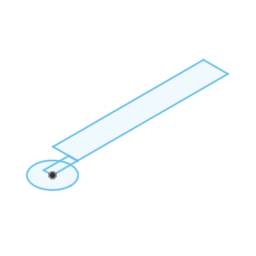
Clip v3 (Autodesk Fusion 360 design; units mm, degrees)
Autodesk Fusion 360 part; units mm, degrees
note: some values were not read from the file. Set by a fixed rule: which sketch regions a step uses.
sketch "Sketch1" plane through (0, 0, 0) normal (0, 0, 1) x (1, 0, 0)
  line L0 (-12.975, 51.3784) -> (12.425, 51.3784)
  line L1 (12.425, 51.3784) -> (12.425, -50.2216)
  line L2 (12.425, -50.2216) -> (-12.975, -50.2216)
  line L3 (-12.975, -50.2216) -> (-12.975, 51.3784)
  line L4 (-0.275, 51.3784) -> (-0.275, -50.2216)
  circle A0 centre (-0.275, -37.535) radius 12.6866
  dimension "d1" = 25.4
  dimension "d2" = 101.6
  constraint horizontal L0
  constraint vertical L1
  constraint horizontal L2
  constraint vertical L3
  constraint midpoint L0 L4.start
  constraint midpoint L2 L4.end
  constraint coincident L4 A0.centre
  constraint coincident L4.end A0
  measures "d1" distance of L0.start L0.end
  measures "d2" distance of L0.start L2.end
extrude "Extrude1" add sketch "Sketch1" along normal blind 25.4 contours L0 L1 L2 L4 A0 | L4 A0 | L4 A0 makes body 1
sketch "Sketch2" plane through (0, 0, 0) normal (0, 0, 1) x (1, 0, 0)
  line L0 (-12.6711, 51.3224) -> (-0.3089, 51.3224)
  line L1 (-0.3089, 51.3224) -> (-0.3089, -24.9086)
  line L2 (-0.3089, -24.9086) -> (-12.6711, -24.9086)
  line L3 (-12.6711, -24.9086) -> (-12.6711, 51.3224)
  circle A0 centre (-0.2821, -37.5504) radius 9.1745
  line L4 (-4.7108, -24.9086) -> (-0.2821, -24.9086)
  line L5 (-0.2821, -24.9086) -> (-0.2821, -37.5504)
  line L6 (-0.2821, -37.5504) -> (-4.7108, -37.5504)
  line L7 (-4.7108, -37.5504) -> (-4.7108, -24.9086)
  constraint horizontal L0
  constraint vertical L1
  constraint horizontal L2
  constraint vertical L3
  constraint horizontal L4
  constraint vertical L5
  constraint horizontal L6
  constraint vertical L7
  constraint coincident A0.centre L5.end
  constraint coincident L2 L4.start
extrude "Extrude2" add sketch "Sketch2" along normal blind 25.4 separate body makes body 2
extrude "Extrude3" cut sketch "Sketch2" along normal blind 261.62 contours A0 L5 L6 L7 | A0 L5 L6 L7 bodies 1
sketch "Sketch3" plane through (0, 0, 25.4) normal (0, 0, 1) x (-1, 0, 0)
  line L0 (4.7108, 24.9086) -> (4.7108, 29.5156)
  arc A0 (4.7108, 29.5156) -> (0.2821, 28.3759) centre (0.2821, 37.5504) ccw
  line L1 (0.2821, 28.3759) -> (0.2821, 24.9086)
  line L2 (0.2821, 24.9086) -> (0.3089, 24.9086)
  line L3 (0.3089, 24.9086) -> (0.3089, -51.3224)
  line L4 (0.3089, -51.3224) -> (12.6711, -51.3224)
  line L5 (12.6711, -51.3224) -> (12.6711, 24.9086)
  line L6 (12.6711, 24.9086) -> (4.7108, 24.9086)
  line L7 (0.3089, 24.9086) -> (4.7108, 24.9086)
  line L8 (0.2821, 28.3759) -> (4.7108, 29.5156)
  constraint coincident L2.end L3.start
  constraint coincident L0.start L6.end
  constraint coincident A0.end L1.start
  constraint coincident L0.end A0.start
extrude "Extrude4" cut sketch "Sketch3" against normal blind 5.08 contours L0 L1 L2 L7 L8 bodies 2
sketch "Sketch4" plane through (0, 0, 0) normal (0, 0, -1) x (1, 0, 0)
  line L0 (-4.7108, 29.5156) -> (-4.7108, 24.9086)
  line L1 (-4.7108, 24.9086) -> (-12.6711, 24.9086)
  line L2 (-12.6711, 24.9086) -> (-12.6711, -51.3224)
  line L3 (-12.6711, -51.3224) -> (-0.3089, -51.3224)
  line L4 (-0.3089, -51.3224) -> (-0.3089, 24.9086)
  line L5 (-0.3089, 24.9086) -> (-0.2821, 24.9086)
  line L6 (-0.2821, 24.9086) -> (-0.2821, 28.3759)
  arc A0 (-0.2821, 28.3759) -> (-4.7108, 29.5156) centre (-0.2821, 37.5504) ccw
  line L7 (-4.7108, 29.5156) -> (-0.2821, 28.3759)
  line L8 (-0.3089, 24.9086) -> (-4.7108, 24.9086)
  constraint coincident L0.start A0.end
  constraint coincident L6.end A0.start
  constraint coincident L4.end L5.start
  constraint coincident L0.end L1.start
extrude "Extrude5" cut sketch "Sketch4" against normal blind 5.08 contours L0 L5 L6 L7 L8 bodies 2
ref_plane "WorkPlane1" through (-12.9616, -37.535, 13.4339) normal (-1, 0, 0) x (0, 1, 0)
sketch "Sketch5" plane through (-12.9616, -37.535, 13.4339) normal (-1, 0, 0) x (0, 1, 0)
  line L0 (12.5644, -7.0697) -> (-9.3081, -7.0697)
  line L1 (-9.3081, -7.0697) -> (-9.3081, 8.3746)
  line L2 (-9.3081, 8.3746) -> (12.5644, 8.3746)
  line L3 (12.5644, 8.3746) -> (12.5644, -7.0697)
  constraint horizontal L0
  constraint vertical L1
  constraint horizontal L2
  constraint vertical L3
extrude "Extrude6" cut sketch "Sketch5" against normal blind 10.16 bodies 1
sketch "Sketch6" plane through (0, 0, 25.4) normal (0, 0, 1) x (-1, 0, 0)
  circle A0 centre (0.2821, 37.5504) radius 9.1745
  line L0 (-12.425, -51.3784) -> (0.275, -51.3784)
  line L1 (0.275, -51.3784) -> (0.275, 24.8484)
  arc A1 (0.275, 24.8484) -> (0.275, 50.2216) centre (0.275, 37.535) ccw
  line L2 (0.275, 50.2216) -> (-12.425, 50.2216)
  line L3 (-12.425, 50.2216) -> (-12.425, -51.3784)
  line L4 (-12.425, -51.3784) -> (-12.425, -56.9551)
  line L5 (-12.425, -56.9551) -> (17.6379, -56.9551)
  line L6 (17.6379, -56.9551) -> (12.8362, -43.9046)
  line L7 (12.8362, -43.9046) -> (12.8362, -51.5381)
  line L8 (12.8362, -51.5381) -> (-12.425, -51.3784)
  constraint coincident L0.start L3.end
  constraint perpendicular L0 L4
  constraint perpendicular L4 L5
  constraint parallel L4 L7
extrude "Extrude7" add sketch "Sketch6" against normal blind 25.4 separate body contours L4 L5 L6 L7 L8 makes body 3
combine "Combine1" operation add target body 1 tool bodies 3
copy_body "Body->Comp1" bodies 1 removing the originals makes body 4 in component "Component"
copy_body "Body->Comp2" bodies 2 removing the originals makes body 5 in component "Component'"
component "Component" placed x (1, 0, 0) y (0, 1, 0) z (0, 0, 1) at (0, 0, 0)
component "Component'" placed x (0.173648, 0.984808, 0) y (-0.984808, 0.173648, 0) z (0, 0, 1) at (-37.2131, -30.752, 0)
